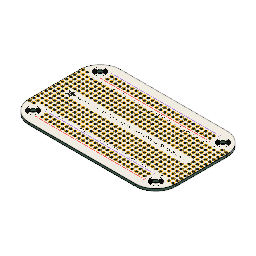
723 Minty Perma-Proto (Autodesk Fusion 360 design; units mm, degrees)
Autodesk Fusion 360 part; units mm, degrees
sketch "Border" plane through (0, 0, 0) normal (0, 1, 0) x (1, 0, 0)
  line L0 (-33.02, 28.448) -> (33.02, 28.448)
  arc A0 (-45.72, 15.748) -> (-33.02, 28.448) centre (-33.02, 15.748) cw
  line L1 (-45.72, -15.748) -> (-45.72, 15.748)
  line L2 (45.72, 15.748) -> (45.72, -15.748)
  line L3 (33.02, -28.448) -> (-33.02, -28.448)
  arc A1 (33.02, 28.448) -> (45.72, 15.748) centre (33.02, 15.748) cw
  arc A2 (45.72, -15.748) -> (33.02, -28.448) centre (33.02, -15.748) cw
  arc A3 (-33.02, -28.448) -> (-45.72, -15.748) centre (-33.02, -15.748) cw
sketch "Holes" plane through (0, 0, 0) normal (0, 1, 0) x (1, 0, 0)
  circle A0 centre (34.29, 8.89) radius 0.6
  circle A1 centre (-8.89, -11.43) radius 0.6
  circle A2 centre (-1.27, -11.43) radius 0.6
  circle A3 centre (-3.81, -3.81) radius 0.6
  circle A4 centre (-1.27, -3.81) radius 0.6
  circle A5 centre (-1.27, -6.35) radius 0.6
  circle A6 centre (1.27, -13.97) radius 0.6
  circle A7 centre (1.27, -11.43) radius 0.6
  circle A8 centre (36.83, 11.43) radius 0.6
  circle A9 centre (-13.97, -6.35) radius 0.6
  circle A10 centre (24.13, -3.81) radius 0.6
  circle A11 centre (34.29, 11.43) radius 0.6
  circle A12 centre (16.51, -13.97) radius 0.6
  circle A13 centre (31.75, -6.35) radius 0.6
  circle A14 centre (34.29, -8.89) radius 0.6
  circle A15 centre (34.29, -13.97) radius 0.6
  circle A16 centre (29.21, -6.35) radius 0.6
  circle A17 centre (19.05, -3.81) radius 0.6
  circle A18 centre (36.83, 13.97) radius 0.6
  circle A19 centre (19.05, -8.89) radius 0.6
  circle A20 centre (29.21, -3.81) radius 0.6
  circle A21 centre (26.67, -11.43) radius 0.6
  circle A22 centre (31.75, 6.35) radius 0.6
  circle A23 centre (16.51, -11.43) radius 0.6
  circle A24 centre (21.59, -3.81) radius 0.6
  circle A25 centre (13.97, -6.35) radius 0.6
  circle A26 centre (34.29, -6.35) radius 0.6
  circle A27 centre (36.83, 8.89) radius 0.6
  circle A28 centre (26.67, -6.35) radius 0.6
  circle A29 centre (19.05, -13.97) radius 0.6
  circle A30 centre (-6.35, -8.89) radius 0.6
  circle A31 centre (8.89, -6.35) radius 0.6
  circle A32 centre (11.43, -13.97) radius 0.6
  circle A33 centre (-16.51, -6.35) radius 0.6
  circle A34 centre (11.43, -11.43) radius 0.6
  circle A35 centre (-21.59, -8.89) radius 0.6
  circle A36 centre (11.43, -8.89) radius 0.6
  circle A37 centre (1.27, -8.89) radius 0.6
  circle A38 centre (6.35, -3.81) radius 0.6
  circle A39 centre (-21.59, -11.43) radius 0.6
  circle A40 centre (-13.97, -13.97) radius 0.6
  circle A41 centre (-19.05, -13.97) radius 0.6
  circle A42 centre (-13.97, -11.43) radius 0.6
  circle A43 centre (-3.81, -13.97) radius 0.6
  circle A44 centre (-16.51, -3.81) radius 0.6
  circle A45 centre (-21.59, -3.81) radius 0.6
  circle A46 centre (6.35, -6.35) radius 0.6
  circle A47 centre (1.27, -3.81) radius 0.6
  circle A48 centre (-8.89, -3.81) radius 0.6
  circle A49 centre (-11.43, -8.89) radius 0.6
  circle A50 centre (-8.89, -8.89) radius 0.6
  circle A51 centre (-8.89, -6.35) radius 0.6
  circle A52 centre (3.81, -6.35) radius 0.6
  circle A53 centre (8.89, -11.43) radius 0.6
  circle A54 centre (3.81, -13.97) radius 0.6
  circle A55 centre (-6.35, -11.43) radius 0.6
  circle A56 centre (-11.43, -13.97) radius 0.6
  circle A57 centre (-6.35, -13.97) radius 0.6
  circle A58 centre (-16.51, -8.89) radius 0.6
  circle A59 centre (-3.81, -11.43) radius 0.6
  circle A60 centre (-1.27, -13.97) radius 0.6
  circle A61 centre (1.27, -6.35) radius 0.6
  circle A62 centre (3.81, -3.81) radius 0.6
  circle A63 centre (3.81, -11.43) radius 0.6
  circle A64 centre (8.89, -13.97) radius 0.6
  circle A65 centre (6.35, -8.89) radius 0.6
  circle A66 centre (31.75, -8.89) radius 0.6
  circle A67 centre (21.59, -6.35) radius 0.6
  circle A68 centre (24.13, -11.43) radius 0.6
  circle A69 centre (36.83, -8.89) radius 0.6
  circle A70 centre (29.21, -11.43) radius 0.6
  circle A71 centre (36.83, -6.35) radius 0.6
  circle A72 centre (36.83, 3.81) radius 0.6
  circle A73 centre (34.29, 13.97) radius 0.6
  circle A74 centre (21.59, -8.89) radius 0.6
  circle A75 centre (31.75, -3.81) radius 0.6
  circle A76 centre (13.97, -11.43) radius 0.6
  circle A77 centre (13.97, -13.97) radius 0.6
  circle A78 centre (26.67, -3.81) radius 0.6
  circle A79 centre (26.67, -8.89) radius 0.6
  circle A80 centre (16.51, -8.89) radius 0.6
  circle A81 centre (16.51, -6.35) radius 0.6
  circle A82 centre (34.29, -11.43) radius 0.6
  circle A83 centre (21.59, -11.43) radius 0.6
  circle A84 centre (24.13, -13.97) radius 0.6
  circle A85 centre (29.21, -13.97) radius 0.6
  circle A86 centre (31.75, -11.43) radius 0.6
  circle A87 centre (21.59, -13.97) radius 0.6
  circle A88 centre (24.13, -8.89) radius 0.6
  circle A89 centre (34.29, -3.81) radius 0.6
  circle A90 centre (13.97, -3.81) radius 0.6
  circle A91 centre (31.75, -13.97) radius 0.6
  circle A92 centre (36.83, -13.97) radius 0.6
  circle A93 centre (13.97, -8.89) radius 0.6
  circle A94 centre (36.83, -3.81) radius 0.6
  circle A95 centre (13.97, 6.35) radius 0.6
  circle A96 centre (29.21, 11.43) radius 0.6
  circle A97 centre (29.21, 13.97) radius 0.6
  circle A98 centre (6.35, 6.35) radius 0.6
  circle A99 centre (29.21, 8.89) radius 0.6
  circle A100 centre (24.13, 8.89) radius 0.6
  circle A101 centre (21.59, 8.89) radius 0.6
  circle A102 centre (24.13, 3.81) radius 0.6
  circle A103 centre (19.05, 8.89) radius 0.6
  circle A104 centre (16.51, 6.35) radius 0.6
  circle A105 centre (13.97, 11.43) radius 0.6
  circle A106 centre (16.51, 8.89) radius 0.6
  circle A107 centre (11.43, 13.97) radius 0.6
  circle A108 centre (19.05, 6.35) radius 0.6
  circle A109 centre (13.97, 13.97) radius 0.6
  circle A110 centre (21.59, 6.35) radius 0.6
  circle A111 centre (8.89, 11.43) radius 0.6
  circle A112 centre (6.35, 11.43) radius 0.6
  circle A113 centre (6.35, 8.89) radius 0.6
  circle A114 centre (24.13, 6.35) radius 0.6
  circle A115 centre (19.05, 13.97) radius 0.6
  circle A116 centre (3.81, 13.97) radius 0.6
  circle A117 centre (3.81, 6.35) radius 0.6
  circle A118 centre (31.75, 3.81) radius 0.6
  circle A119 centre (29.21, 6.35) radius 0.6
  circle A120 centre (26.67, 13.97) radius 0.6
  circle A121 centre (8.89, 3.81) radius 0.6
  circle A122 centre (3.81, 3.81) radius 0.6
  circle A123 centre (21.59, 11.43) radius 0.6
  circle A124 centre (11.43, 8.89) radius 0.6
  circle A125 centre (11.43, 11.43) radius 0.6
  circle A126 centre (21.59, 3.81) radius 0.6
  circle A127 centre (16.51, 13.97) radius 0.6
  circle A128 centre (24.13, 11.43) radius 0.6
  circle A129 centre (13.97, 8.89) radius 0.6
  circle A130 centre (29.21, 3.81) radius 0.6
  circle A131 centre (19.05, 3.81) radius 0.6
  circle A132 centre (3.81, 11.43) radius 0.6
  circle A133 centre (26.67, 3.81) radius 0.6
  circle A134 centre (11.43, 3.81) radius 0.6
  circle A135 centre (6.35, 13.97) radius 0.6
  circle A136 centre (26.67, 11.43) radius 0.6
  circle A137 centre (8.89, 8.89) radius 0.6
  circle A138 centre (1.27, 6.35) radius 0.6
  circle A139 centre (8.89, -21.59) radius 0.6
  circle A140 centre (-8.89, 21.59) radius 0.6
  circle A141 centre (-24.13, -21.59) radius 0.6
  circle A142 centre (29.21, -19.05) radius 0.6
  circle A143 centre (29.21, 21.59) radius 0.6
  circle A144 centre (-31.75, -21.59) radius 0.6
  circle A145 centre (-29.21, -19.05) radius 0.6
  circle A146 centre (-26.67, -21.59) radius 0.6
  circle A147 centre (13.97, 21.59) radius 0.6
  circle A148 centre (26.67, -21.59) radius 0.6
  circle A149 centre (1.27, -21.59) radius 0.6
  circle A150 centre (-13.97, 3.81) radius 0.6
  circle A151 centre (13.97, -19.05) radius 0.6
  circle A152 centre (31.75, -21.59) radius 0.6
  circle A153 centre (21.59, -19.05) radius 0.6
  circle A154 centre (24.13, -19.05) radius 0.6
  circle A155 centre (13.97, -21.59) radius 0.6
  circle A156 centre (16.51, 21.59) radius 0.6
  circle A157 centre (-34.29, 13.97) radius 0.6
  circle A158 centre (11.43, 21.59) radius 0.6
  circle A159 centre (3.81, 21.59) radius 0.6
  circle A160 centre (-11.43, 21.59) radius 0.6
  circle A161 centre (-11.43, -21.59) radius 0.6
  circle A162 centre (-34.29, 11.43) radius 0.6
  circle A163 centre (-29.21, -21.59) radius 0.6
  circle A164 centre (-16.51, 21.59) radius 0.6
  circle A165 centre (-6.35, 21.59) radius 0.6
  circle A166 centre (-13.97, 21.59) radius 0.6
  circle A167 centre (-16.51, -21.59) radius 0.6
  circle A168 centre (19.05, -21.59) radius 0.6
  circle A169 centre (19.05, 21.59) radius 0.6
  circle A170 centre (16.51, -21.59) radius 0.6
  circle A171 centre (6.35, -21.59) radius 0.6
  circle A172 centre (21.59, -21.59) radius 0.6
  circle A173 centre (-29.21, 21.59) radius 0.6
  circle A174 centre (8.89, 21.59) radius 0.6
  circle A175 centre (-21.59, -21.59) radius 0.6
  circle A176 centre (16.51, -19.05) radius 0.6
  circle A177 centre (21.59, 21.59) radius 0.6
  circle A178 centre (6.35, 21.59) radius 0.6
  circle A179 centre (1.27, 21.59) radius 0.6
  circle A180 centre (-31.75, 21.59) radius 0.6
  circle A181 centre (-1.27, 21.59) radius 0.6
  circle A182 centre (-26.67, 21.59) radius 0.6
  circle A183 centre (26.67, 21.59) radius 0.6
  circle A184 centre (-1.27, -21.59) radius 0.6
  circle A185 centre (24.13, 21.59) radius 0.6
  circle A186 centre (3.81, -21.59) radius 0.6
  circle A187 centre (-3.81, 21.59) radius 0.6
  circle A188 centre (-3.81, -21.59) radius 0.6
  circle A189 centre (-41.91, -13.97) radius 0.6
  circle A190 centre (19.05, 19.05) radius 0.6
  circle A191 centre (26.67, -19.05) radius 0.6
  circle A192 centre (-6.35, -21.59) radius 0.6
  circle A193 centre (-19.05, 21.59) radius 0.6
  circle A194 centre (29.21, -21.59) radius 0.6
  circle A195 centre (21.59, 19.05) radius 0.6
  circle A196 centre (31.75, 19.05) radius 0.6
  circle A197 centre (19.05, -19.05) radius 0.6
  circle A198 centre (24.13, -21.59) radius 0.6
  circle A199 centre (-21.59, 21.59) radius 0.6
  circle A200 centre (-24.13, 21.59) radius 0.6
  circle A201 centre (29.21, 19.05) radius 0.6
  circle A202 centre (24.13, 19.05) radius 0.6
  circle A203 centre (-19.05, -21.59) radius 0.6
  circle A204 centre (11.43, -21.59) radius 0.6
  circle A205 centre (26.67, 19.05) radius 0.6
  circle A206 centre (11.43, -19.05) radius 0.6
  circle A207 centre (31.75, 21.59) radius 0.6
  circle A208 centre (-13.97, -21.59) radius 0.6
  circle A209 centre (-8.89, -21.59) radius 0.6
  circle A210 centre (-41.91, -3.81) radius 0.6
  circle A211 centre (-44.45, 8.89) radius 0.6
  circle A212 centre (-39.37, 3.81) radius 0.6
  circle A213 centre (-19.05, 19.05) radius 0.6
  circle A214 centre (-39.37, 8.89) radius 0.6
  circle A215 centre (-41.91, -1.27) radius 0.6
  circle A216 centre (16.51, 19.05) radius 0.6
  circle A217 centre (-39.37, -6.35) radius 0.6
  circle A218 centre (-29.21, 19.05) radius 0.6
  circle A219 centre (-44.45, 6.35) radius 0.6
  circle A220 centre (-41.91, 11.43) radius 0.6
  circle A221 centre (-13.97, 19.05) radius 0.6
  circle A222 centre (-44.45, 3.81) radius 0.6
  circle A223 centre (-6.35, 19.05) radius 0.6
  circle A224 centre (-39.37, 6.35) radius 0.6
  circle A225 centre (-31.75, 19.05) radius 0.6
  circle A226 centre (8.89, 19.05) radius 0.6
  circle A227 centre (-16.51, 19.05) radius 0.6
  circle A228 centre (-3.81, 19.05) radius 0.6
  circle A229 centre (-44.45, 13.97) radius 0.6
  circle A230 centre (-41.91, 1.27) radius 0.6
  circle A231 centre (-44.45, -6.35) radius 0.6
  circle A232 centre (-11.43, 19.05) radius 0.6
  circle A233 centre (-8.89, 19.05) radius 0.6
  circle A234 centre (-44.45, -1.27) radius 0.6
  circle A235 centre (-44.45, 11.43) radius 0.6
  circle A236 centre (-39.37, -13.97) radius 0.6
  circle A237 centre (-44.45, -8.89) radius 0.6
  circle A238 centre (11.43, 19.05) radius 0.6
  circle A239 centre (-44.45, -11.43) radius 0.6
  circle A240 centre (-41.91, 16.51) radius 0.6
  circle A241 centre (6.35, 19.05) radius 0.6
  circle A242 centre (-41.91, 6.35) radius 0.6
  circle A243 centre (-41.91, -6.35) radius 0.6
  circle A244 centre (-41.91, 3.81) radius 0.6
  circle A245 centre (-39.37, -11.43) radius 0.6
  circle A246 centre (-44.45, 16.51) radius 0.6
  circle A247 centre (-41.91, -11.43) radius 0.6
  circle A248 centre (-39.37, -3.81) radius 0.6
  circle A249 centre (-44.45, -3.81) radius 0.6
  circle A250 centre (13.97, 19.05) radius 0.6
  circle A251 centre (-1.27, 19.05) radius 0.6
  circle A252 centre (-39.37, 1.27) radius 0.6
  circle A253 centre (-26.67, 19.05) radius 0.6
  circle A254 centre (-41.91, 8.89) radius 0.6
  circle A255 centre (-39.37, 11.43) radius 0.6
  circle A256 centre (-41.91, 13.97) radius 0.6
  circle A257 centre (-39.37, -8.89) radius 0.6
  circle A258 centre (-39.37, 13.97) radius 0.6
  circle A259 centre (-41.91, -8.89) radius 0.6
  circle A260 centre (1.27, 19.05) radius 0.6
  circle A261 centre (-24.13, 19.05) radius 0.6
  circle A262 centre (-44.45, 1.27) radius 0.6
  circle A263 centre (41.91, 16.51) radius 0.6
  circle A264 centre (41.91, -16.51) radius 0.6
  circle A265 centre (-44.45, -16.51) radius 0.6
  circle A266 centre (39.37, -1.27) radius 0.6
  circle A267 centre (38.1, -20.828) radius 1.5
  circle A268 centre (-44.45, -13.97) radius 0.6
  circle A269 centre (44.45, 13.97) radius 0.6
  circle A270 centre (41.91, -13.97) radius 0.6
  circle A271 centre (39.37, 11.43) radius 0.6
  circle A272 centre (-41.91, -16.51) radius 0.6
  circle A273 centre (-39.37, -1.27) radius 0.6
  circle A274 centre (39.37, 13.97) radius 0.6
  circle A275 centre (3.81, 19.05) radius 0.6
  circle A276 centre (39.37, 8.89) radius 0.6
  circle A277 centre (41.91, 1.27) radius 0.6
  circle A278 centre (-21.59, 19.05) radius 0.6
  circle A279 centre (-38.1, 20.828) radius 1.5
  circle A280 centre (41.91, 8.89) radius 0.6
  circle A281 centre (-38.1, -20.828) radius 1.5
  circle A282 centre (44.45, -8.89) radius 0.6
  circle A283 centre (41.91, -11.43) radius 0.6
  circle A284 centre (41.91, 11.43) radius 0.6
  circle A285 centre (41.91, 6.35) radius 0.6
  circle A286 centre (44.45, 11.43) radius 0.6
  circle A287 centre (41.91, -1.27) radius 0.6
  circle A288 centre (44.45, -3.81) radius 0.6
  circle A289 centre (38.1, 20.828) radius 1.5
  circle A290 centre (41.91, 13.97) radius 0.6
  circle A291 centre (44.45, 8.89) radius 0.6
  circle A292 centre (44.45, -6.35) radius 0.6
  circle A293 centre (44.45, -13.97) radius 0.6
  circle A294 centre (41.91, -8.89) radius 0.6
  circle A295 centre (39.37, -3.81) radius 0.6
  circle A296 centre (39.37, -8.89) radius 0.6
  circle A297 centre (44.45, 6.35) radius 0.6
  circle A298 centre (39.37, 1.27) radius 0.6
  circle A299 centre (41.91, 3.81) radius 0.6
  circle A300 centre (-29.21, -13.97) radius 0.6
  circle A301 centre (-36.83, -3.81) radius 0.6
  circle A302 centre (41.91, -3.81) radius 0.6
  circle A303 centre (-19.05, -11.43) radius 0.6
  circle A304 centre (-24.13, -11.43) radius 0.6
  circle A305 centre (-34.29, -13.97) radius 0.6
  circle A306 centre (-19.05, -6.35) radius 0.6
  circle A307 centre (41.91, -6.35) radius 0.6
  circle A308 centre (39.37, -11.43) radius 0.6
  circle A309 centre (44.45, -1.27) radius 0.6
  circle A310 centre (39.37, 3.81) radius 0.6
  circle A311 centre (-29.21, -11.43) radius 0.6
  circle A312 centre (-26.67, -11.43) radius 0.6
  circle A313 centre (44.45, -11.43) radius 0.6
  circle A314 centre (-36.83, -11.43) radius 0.6
  circle A315 centre (-29.21, -3.81) radius 0.6
  circle A316 centre (-24.13, -3.81) radius 0.6
  circle A317 centre (-29.21, -8.89) radius 0.6
  circle A318 centre (44.45, 16.51) radius 0.6
  circle A319 centre (44.45, 1.27) radius 0.6
  circle A320 centre (-19.05, -8.89) radius 0.6
  circle A321 centre (-31.75, -6.35) radius 0.6
  circle A322 centre (-34.29, -8.89) radius 0.6
  circle A323 centre (39.37, 6.35) radius 0.6
  circle A324 centre (-36.83, -6.35) radius 0.6
  circle A325 centre (-31.75, -3.81) radius 0.6
  circle A326 centre (-31.75, -8.89) radius 0.6
  circle A327 centre (44.45, -16.51) radius 0.6
  circle A328 centre (-36.83, -13.97) radius 0.6
  circle A329 centre (39.37, -6.35) radius 0.6
  circle A330 centre (-26.67, -13.97) radius 0.6
  circle A331 centre (-31.75, -13.97) radius 0.6
  circle A332 centre (-26.67, -8.89) radius 0.6
  circle A333 centre (-26.67, -6.35) radius 0.6
  circle A334 centre (-31.75, -11.43) radius 0.6
  circle A335 centre (-19.05, -3.81) radius 0.6
  circle A336 centre (39.37, -13.97) radius 0.6
  circle A337 centre (-24.13, -6.35) radius 0.6
  circle A338 centre (-24.13, -8.89) radius 0.6
  circle A339 centre (-29.21, -6.35) radius 0.6
  circle A340 centre (-34.29, -11.43) radius 0.6
  circle A341 centre (-24.13, -13.97) radius 0.6
  circle A342 centre (-26.67, -3.81) radius 0.6
  circle A343 centre (-34.29, -6.35) radius 0.6
  circle A344 centre (-34.29, -3.81) radius 0.6
  circle A345 centre (-36.83, -8.89) radius 0.6
  circle A346 centre (-21.59, -13.97) radius 0.6
  circle A347 centre (44.45, 3.81) radius 0.6
  circle A348 centre (1.27, -19.05) radius 0.6
  circle A349 centre (-34.29, 6.35) radius 0.6
  circle A350 centre (-26.67, 8.89) radius 0.6
  circle A351 centre (-26.67, 11.43) radius 0.6
  circle A352 centre (-19.05, 6.35) radius 0.6
  circle A353 centre (-31.75, 3.81) radius 0.6
  circle A354 centre (-26.67, 6.35) radius 0.6
  circle A355 centre (-19.05, 11.43) radius 0.6
  circle A356 centre (-24.13, 11.43) radius 0.6
  circle A357 centre (-13.97, 8.89) radius 0.6
  circle A358 centre (-31.75, 11.43) radius 0.6
  circle A359 centre (-8.89, -19.05) radius 0.6
  circle A360 centre (-19.05, 13.97) radius 0.6
  circle A361 centre (-21.59, -19.05) radius 0.6
  circle A362 centre (-19.05, -19.05) radius 0.6
  circle A363 centre (-13.97, 13.97) radius 0.6
  circle A364 centre (-21.59, 3.81) radius 0.6
  circle A365 centre (-19.05, 8.89) radius 0.6
  circle A366 centre (-1.27, -19.05) radius 0.6
  circle A367 centre (-31.75, -19.05) radius 0.6
  circle A368 centre (-36.83, 13.97) radius 0.6
  circle A369 centre (-13.97, 6.35) radius 0.6
  circle A370 centre (-24.13, 8.89) radius 0.6
  circle A371 centre (-31.75, 6.35) radius 0.6
  circle A372 centre (-29.21, 6.35) radius 0.6
  circle A373 centre (-29.21, 13.97) radius 0.6
  circle A374 centre (-19.05, 3.81) radius 0.6
  circle A375 centre (-6.35, -19.05) radius 0.6
  circle A376 centre (-16.51, -19.05) radius 0.6
  circle A377 centre (-34.29, 3.81) radius 0.6
  circle A378 centre (-13.97, -19.05) radius 0.6
  circle A379 centre (-29.21, 11.43) radius 0.6
  circle A380 centre (-34.29, 8.89) radius 0.6
  circle A381 centre (-26.67, 3.81) radius 0.6
  circle A382 centre (-24.13, -19.05) radius 0.6
  circle A383 centre (-31.75, 8.89) radius 0.6
  circle A384 centre (-26.67, 13.97) radius 0.6
  circle A385 centre (-36.83, 6.35) radius 0.6
  circle A386 centre (-36.83, 3.81) radius 0.6
  circle A387 centre (-21.59, 11.43) radius 0.6
  circle A388 centre (-24.13, 3.81) radius 0.6
  circle A389 centre (-26.67, -19.05) radius 0.6
  circle A390 centre (-31.75, 13.97) radius 0.6
  circle A391 centre (-11.43, -19.05) radius 0.6
  circle A392 centre (-21.59, 13.97) radius 0.6
  circle A393 centre (-36.83, 11.43) radius 0.6
  circle A394 centre (-29.21, 3.81) radius 0.6
  circle A395 centre (-36.83, 8.89) radius 0.6
  circle A396 centre (-29.21, 8.89) radius 0.6
  circle A397 centre (-21.59, 8.89) radius 0.6
  circle A398 centre (-13.97, 11.43) radius 0.6
  circle A399 centre (31.75, -19.05) radius 0.6
  circle A400 centre (6.35, -19.05) radius 0.6
  circle A401 centre (-21.59, 6.35) radius 0.6
  circle A402 centre (8.89, -19.05) radius 0.6
  circle A403 centre (-3.81, -19.05) radius 0.6
  circle A404 centre (-24.13, 6.35) radius 0.6
  circle A405 centre (-24.13, 13.97) radius 0.6
  circle A406 centre (3.81, -19.05) radius 0.6
  circle A407 centre (36.83, -11.43) radius 0.6
  circle A408 centre (36.83, 6.35) radius 0.6
  circle A409 centre (31.75, 11.43) radius 0.6
  circle A410 centre (31.75, 8.89) radius 0.6
  circle A411 centre (34.29, 6.35) radius 0.6
  circle A412 centre (34.29, 3.81) radius 0.6
  circle A413 centre (31.75, 13.97) radius 0.6
  circle A414 centre (19.05, -11.43) radius 0.6
  circle A415 centre (26.67, -13.97) radius 0.6
  circle A416 centre (16.51, -3.81) radius 0.6
  circle A417 centre (24.13, -6.35) radius 0.6
  circle A418 centre (19.05, -6.35) radius 0.6
  circle A419 centre (29.21, -8.89) radius 0.6
  circle A420 centre (-16.51, -13.97) radius 0.6
  circle A421 centre (-16.51, -11.43) radius 0.6
  circle A422 centre (8.89, -3.81) radius 0.6
  circle A423 centre (-8.89, -13.97) radius 0.6
  circle A424 centre (-3.81, -8.89) radius 0.6
  circle A425 centre (-3.81, -6.35) radius 0.6
  circle A426 centre (-13.97, -3.81) radius 0.6
  circle A427 centre (6.35, -13.97) radius 0.6
  circle A428 centre (-1.27, -8.89) radius 0.6
  circle A429 centre (3.81, -8.89) radius 0.6
  circle A430 centre (-6.35, -6.35) radius 0.6
  circle A431 centre (8.89, -8.89) radius 0.6
  circle A432 centre (-11.43, -6.35) radius 0.6
  circle A433 centre (6.35, -11.43) radius 0.6
  circle A434 centre (11.43, -6.35) radius 0.6
  circle A435 centre (11.43, -3.81) radius 0.6
  circle A436 centre (-6.35, -3.81) radius 0.6
  circle A437 centre (-21.59, -6.35) radius 0.6
  circle A438 centre (-13.97, -8.89) radius 0.6
  circle A439 centre (-11.43, -3.81) radius 0.6
  circle A440 centre (-11.43, -11.43) radius 0.6
  circle A441 centre (-6.35, 3.81) radius 0.6
  circle A442 centre (-6.35, 6.35) radius 0.6
  circle A443 centre (-16.51, 13.97) radius 0.6
  circle A444 centre (-8.89, 11.43) radius 0.6
  circle A445 centre (-3.81, 11.43) radius 0.6
  circle A446 centre (-16.51, 11.43) radius 0.6
  circle A447 centre (-8.89, 6.35) radius 0.6
  circle A448 centre (-8.89, 8.89) radius 0.6
  circle A449 centre (-8.89, 13.97) radius 0.6
  circle A450 centre (-3.81, 13.97) radius 0.6
  circle A451 centre (-11.43, 6.35) radius 0.6
  circle A452 centre (-3.81, 8.89) radius 0.6
  circle A453 centre (-3.81, 6.35) radius 0.6
  circle A454 centre (-11.43, 13.97) radius 0.6
  circle A455 centre (-6.35, 13.97) radius 0.6
  circle A456 centre (-16.51, 8.89) radius 0.6
  circle A457 centre (-16.51, 6.35) radius 0.6
  circle A458 centre (-1.27, 3.81) radius 0.6
  circle A459 centre (-3.81, 3.81) radius 0.6
  circle A460 centre (-8.89, 3.81) radius 0.6
  circle A461 centre (-6.35, 11.43) radius 0.6
  circle A462 centre (1.27, 13.97) radius 0.6
  circle A463 centre (13.97, 3.81) radius 0.6
  circle A464 centre (-1.27, 13.97) radius 0.6
  circle A465 centre (1.27, 11.43) radius 0.6
  circle A466 centre (21.59, 13.97) radius 0.6
  circle A467 centre (19.05, 11.43) radius 0.6
  circle A468 centre (16.51, 11.43) radius 0.6
  circle A469 centre (16.51, 3.81) radius 0.6
  circle A470 centre (1.27, 8.89) radius 0.6
  circle A471 centre (1.27, 3.81) radius 0.6
  circle A472 centre (8.89, 13.97) radius 0.6
  circle A473 centre (6.35, 3.81) radius 0.6
  circle A474 centre (-1.27, 8.89) radius 0.6
  circle A475 centre (-11.43, 11.43) radius 0.6
  circle A476 centre (-11.43, 8.89) radius 0.6
  circle A477 centre (-1.27, 6.35) radius 0.6
  circle A478 centre (-1.27, 11.43) radius 0.6
  circle A479 centre (8.89, 6.35) radius 0.6
  circle A480 centre (26.67, 6.35) radius 0.6
  circle A481 centre (24.13, 13.97) radius 0.6
  circle A482 centre (-11.43, 3.81) radius 0.6
  circle A483 centre (-6.35, 8.89) radius 0.6
  circle A484 centre (-16.51, 3.81) radius 0.6
  circle A485 centre (26.67, 8.89) radius 0.6
  circle A486 centre (3.81, 8.89) radius 0.6
  circle A487 centre (11.43, 6.35) radius 0.6
extrude "Extrude1" add sketch "Border" along normal blind 1.57
extrude "Extrude2" cut sketch "Holes" along normal blind 1.57
equation "BoardThickness = 1.57 mm"
equation "d2 = BoardThickness"
equation "d4 = BoardThickness"
named bodies: "PCB"
